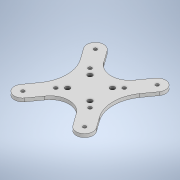
# Autodesk Inventor part: bottom plate
Saved by Autodesk Inventor 2020 (Build 240168000, 168)
## iProperties
Created: 2022-08-17
Part Number: bottom plate
Material: Generic
Document SubType Name: Modeling
Designer: Steven
Density: 1 g/cm^3
Appearance: Default
Author: Steven
Autodesk Inventor part; units mm, degrees
ref_plane "YZ Plane" through (0, 0, 0) normal (1, 0, 0) x (0, 1, 0)
ref_plane "XZ Plane" through (0, 0, 0) normal (0, 1, 0) x (-1, 0, 0)
ref_plane "XY Plane" through (0, 0, 0) normal (0, 0, 1) x (1, 0, 0)
sketch "Sketch1" plane through (0, 0, 0) normal (0, 1, 0) x (-1, 0, 0)
  arc A0 (-2.9502, -0.8481) -> (-2.9502, 0.8481) centre (-3.48, 0) ccw
  line L0 (-2.9502, 0.8481) -> (-7.8639, 3.9177)
  arc A1 (-7.8639, 3.9177) -> (-9.3575, 3.336) centre (-8.3937, 3.0696) ccw
  line L1 (-9.3575, 3.336) -> (-10.206, 0.2664)
  arc A2 (-10.206, 0.2664) -> (-10.206, -0.2664) centre (-9.2421, 0) ccw
  line L2 (-10.206, -0.2664) -> (-9.3575, -3.336)
  arc A3 (-9.3575, -3.336) -> (-7.8639, -3.9177) centre (-8.3937, -3.0696) ccw
  line L3 (-7.8639, -3.9177) -> (-2.9502, -0.8481)
  line L4 (-21.4137, 36.6803) -> (-21.3554, 36.5991)
  line L5 (18.0989, 21.6995) -> (22.3004, 27.5465)
  circle A4 centre (27.5044, 32.3038) radius 1.475
  line L6 (7.8639, 3.9177) -> (2.9502, 0.8481)
  arc A5 (2.9502, 0.8481) -> (2.9502, -0.8481) centre (3.48, 0) ccw
  line L7 (2.9502, -0.8481) -> (7.8639, -3.9177)
  arc A6 (7.8639, -3.9177) -> (9.3575, -3.336) centre (8.3937, -3.0696) ccw
  line L8 (9.3575, -3.336) -> (10.206, -0.2664)
  arc A7 (10.206, -0.2664) -> (10.206, 0.2664) centre (9.2421, 0) ccw
  line L9 (10.206, 0.2664) -> (9.3575, 3.336)
  arc A8 (9.3575, 3.336) -> (7.8639, 3.9177) centre (8.3937, 3.0696) ccw
  line L10 (-24.6555, 25.8542) -> (-20.454, 20.0072)
  arc A9 (-20.454, 20.0072) -> (-18.0989, 21.6995) centre (-19.2764, 20.8534) ccw
  line L11 (-18.0989, 21.6995) -> (-22.3004, 27.5465)
  arc A10 (-22.3004, 27.5465) -> (-24.6555, 25.8542) centre (-23.4779, 26.7004) ccw
  line L12 (14.2256, 26.6769) -> (21.4137, 36.6803)
  arc A11 (-26.3995, -17.9136) -> (-26.3995, 17.9136) centre (-51.8984, 0) ccw
  arc A12 (26.3995, 17.9136) -> (26.3995, -17.9136) centre (51.8984, 0) ccw
  line L13 (-21.3365, 36.5729) -> (-12.8954, 24.8295)
  arc A13 (-12.8954, 24.8295) -> (14.2256, 26.6769) centre (-0.0002, 35.5195) ccw
  arc A14 (18.0989, 21.6995) -> (20.454, 20.0072) centre (19.2764, 20.8534) ccw
  line L14 (24.6555, 25.8542) -> (20.454, 20.0072)
  circle A15 centre (15.2498, 15.25) radius 1.475
  arc A16 (-21.3554, 36.5991) -> (-21.3365, 36.5729) centre (0, 51.9445) ccw
  circle A17 centre (-15.2502, 15.25) radius 1.475
  line L15 (33.595, 27.9272) -> (26.3995, 17.9136)
  arc A18 (24.6555, 25.8542) -> (22.3004, 27.5465) centre (23.4779, 26.7004) ccw
  arc A19 (33.595, 27.9272) -> (21.4137, 36.6803) centre (27.5044, 32.3038) ccw
  line L16 (-22.3004, -27.5465) -> (-18.0989, -21.6995)
  arc A20 (-18.0989, -21.6995) -> (-20.454, -20.0072) centre (-19.2764, -20.8534) ccw
  line L17 (-20.454, -20.0072) -> (-24.6555, -25.8542)
  arc A21 (-24.6555, -25.8542) -> (-22.3004, -27.5465) centre (-23.4779, -26.7004) ccw
  circle A22 centre (10, 10) radius 2.1
  circle A23 centre (-10, 10) radius 2.1
  arc A24 (-21.4137, 36.6803) -> (-33.595, 27.9272) centre (-27.5044, 32.3038) ccw
  line L18 (-26.3995, 17.9136) -> (-33.595, 27.9272)
  circle A25 centre (-27.5044, 32.3038) radius 1.475
  line L19 (-21.3554, -36.5991) -> (-21.4137, -36.6803)
  circle A26 centre (15.2498, -15.25) radius 1.475
  line L20 (18.0989, -21.6995) -> (22.3004, -27.5465)
  arc A27 (22.3004, -27.5465) -> (24.6555, -25.8542) centre (23.4779, -26.7004) ccw
  line L21 (24.6555, -25.8542) -> (20.454, -20.0072)
  arc A28 (20.454, -20.0072) -> (18.0989, -21.6995) centre (19.2764, -20.8534) ccw
  circle A29 centre (27.5044, -32.3038) radius 1.475
  circle A30 centre (-10.0002, -10) radius 2.1
  circle A31 centre (10, -10) radius 2.1
  line L22 (-14.2191, -26.666) -> (-21.3554, -36.5991)
  line L23 (21.3554, -36.5991) -> (14.2318, -26.6869)
  circle A32 centre (-15.2502, -15.25) radius 1.475
  circle A33 centre (-27.5044, -32.3038) radius 1.475
  arc A34 (21.4137, -36.6803) -> (33.595, -27.9272) centre (27.5044, -32.3038) ccw
  line L24 (-33.595, -27.9272) -> (-26.3995, -17.9136)
  arc A35 (14.2318, -26.6869) -> (-14.2191, -26.666) centre (-0.0002, -35.5195) ccw
  line L25 (26.3995, -17.9136) -> (33.595, -27.9272)
  line L26 (21.4137, -36.6803) -> (21.3554, -36.5991)
  arc A36 (-33.595, -27.9272) -> (-21.4137, -36.6803) centre (-27.5044, -32.3038) ccw
  line L27 (3.48, 0) -> (-3.48, 0) construction
  point P0 (0, 0)
  point P1 (0, 0)
  point P2 (-21.4137, 36.6803)
  point P3 (-33.595, 27.9272)
  point P4 (-21.4137, -36.6803)
  point P5 (21.4137, -36.6803)
  point P6 (21.4137, 36.6803)
  point P7 (-12.8954, 24.8295)
  point P8 (-21.3365, 36.5729)
  point P9 (-21.3554, 36.5991)
  constraints: 56 end point, 50 point on circle, 37 centre point, 1 horizontal, 1 midpoint
extrude "Extrusion1" add sketch "Sketch1" along normal blind 3 contours L3 A3 L2 A2 L1 A1 L0 A0 | L4 A16 L13 A13 L12 A19 L15 A12 L25 A34 L26 L23 A35 L22 L19 A36 L24 A11 L18 A24 | L5 A18 L14 A14 | A8 L9 A7 L8 A6 L7 A5 L6 | A10 L11 A9 L10 | A21 L17 A20 L16 | A28 L21 A27 L20
sketch "Sketch2" plane through (0, 3, 0) normal (0, 1, 0) x (1, 0, 0)
  circle A0 centre (-15.2498, 15.25) radius 1.475 construction
  circle A1 centre (15.2502, 15.25) radius 1.475 construction
  circle A2 centre (15.2502, -15.25) radius 1.475 construction
  circle A3 centre (-15.2498, -15.25) radius 1.475 construction
  circle A4 centre (-15.2498, 15.25) radius 1.475 projected
  circle A5 centre (-15.2498, 15.25) radius 1.55
  circle A6 centre (15.2502, 15.25) radius 1.475 projected
  circle A7 centre (15.2502, 15.25) radius 1.55
  circle A8 centre (15.2502, -15.25) radius 1.475 projected
  circle A9 centre (15.2502, -15.25) radius 1.55
  circle A10 centre (-15.2498, -15.25) radius 1.55
  point P0 (0, 0)
  dimension "d2" = 3.1
  dimension "d3" = 3.1
  dimension "d4" = 3.1
  dimension "d5" = 3.1
  constraints: 4 centre point, 4 coincident
  measures "d2" diameter of A5
  measures "d3" diameter of A7
  measures "d4" diameter of A9
  measures "d5" diameter of A10
extrude "Extrusion2" cut sketch "Sketch2" against normal through all contours A4 | A5 | A6 | A7 | A8 | A9 | A10
body "Solid1"
